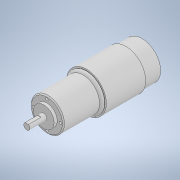
# Autodesk Inventor part: RS-555-71
Saved by Autodesk Inventor 2021 (Build 250183000, 183)
## iProperties
Created: 2022-02-01
Part Number: RS-555-71
Material: 一般
Document SubType Name: Modeling
Designer: hirohumi
Density: 1 g/cm^3
Appearance: 既定
Author: hirohumi
Autodesk Inventor part; units mm, degrees
ref_plane "YZ Plane" through (0, 0, 0) normal (1, 0, 0) x (0, 1, 0)
ref_plane "XZ Plane" through (0, 0, 0) normal (0, 1, 0) x (-1, 0, 0)
ref_plane "XY Plane" through (0, 0, 0) normal (0, 0, 1) x (1, 0, 0)
sketch "スケッチ1" plane through (0, 0, 0) normal (0, 0, 1) x (1, 0, 0)
  circle A0 centre (0, 0) radius 17.9
  dimension "d0" = 35.8
  constraints: 1 centre point, 1 coincident
  measures "d0" diameter of A0
extrude "押し出し1" add sketch "スケッチ1" against normal blind 3.3
fillet "フィレット1" radius 3 1 edges at (-17.9, 0, 0)
sketch "スケッチ2" plane through (0, 0, -3.3) normal (0, 0, -1) x (-1, 0, 0)
  circle A0 centre (0, 0) radius 19.25
  dimension "d4" = 38.5
  constraints: 1 centre point, 1 coincident
  measures "d4" diameter of A0
extrude "押し出し2" add sketch "スケッチ2" along normal blind 38
sketch "スケッチ3" plane through (0, 0, -41.3) normal (0, 0, -1) x (-1, 0, 0)
  circle A0 centre (0, 0) radius 17.9
  dimension "d7" = 35.8
  constraints: 1 centre point, 1 coincident
  measures "d7" diameter of A0
extrude "押し出し3" add sketch "スケッチ3" along normal blind 15.7
sketch "スケッチ4" plane through (0, 0, -57) normal (0, 0, -1) x (-1, 0, 0)
  circle A0 centre (0, 0) radius 1.585
  dimension "d10" = 3.17
  constraints: 1 centre point, 1 coincident
  measures "d10" diameter of A0
extrude "押し出し4" add sketch "スケッチ4" along normal blind 10.7
sketch "スケッチ5" plane through (0, 0, 0) normal (0, 0, 1) x (1, 0, 0)
  circle A0 centre (0, 0) radius 1.585 projected
  circle A1 centre (0, 0) radius 16
  dimension "d13" = 32
  constraints: 1 centre point, 1 coincident
  measures "d13" diameter of A1
extrude "押し出し5" add sketch "スケッチ5" along normal blind 34.9 contours A0 | A1
chamfer "面取り1" distance 1 angle 45 1 edges at (-16, 0, 34.9)
sketch "スケッチ6" plane through (0, 0, 34.9) normal (0, 0, 1) x (1, 0, 0)
  circle A0 centre (0, 0) radius 10
  dimension "d19" = 20
  constraints: 1 centre point, 1 coincident
  measures "d19" diameter of A0
extrude "押し出し6" add sketch "スケッチ6" along normal blind 3
sketch "スケッチ7" plane through (0, 0, 37.9) normal (0, 0, 1) x (1, 0, 0)
  circle A0 centre (0, 0) radius 1.585 projected
  circle A1 centre (0, 0) radius 3
  dimension "d22" = 6
  constraints: 1 centre point, 1 coincident
  measures "d22" diameter of A1
extrude "押し出し7" add sketch "スケッチ7" along normal blind 16.3 contours A0 | A1
sketch "スケッチ8" plane through (0, 0, 54.2) normal (0, 0, 1) x (1, 0, 0)
  circle A0 centre (0, 0) radius 3 projected
  line L0 (-1.6583, 2.5) -> (1.6583, 2.5)
  arc A1 (1.6583, 2.5) -> (-1.6583, 2.5) centre (0, 0) ccw
  dimension "d25" = 2.5
  constraints: 4 point on circle, 2 end point, 1 centre point, 1 coincident, 1 horizontal
  measures "d25" distance from line of point (0, 0) L0
extrude "押し出し8" cut sketch "スケッチ8" against normal blind 12 contours L0 A0 picked at (-0.1169, 2.6598)
sketch "スケッチ9" plane through (0, 0, 34.9) normal (0, 0, 1) x (1, 0, 0)
  circle A0 centre (0, 13) radius 1.25
  circle A1 centre (-13, 0) radius 1.25
  circle A2 centre (0, -13) radius 1.25
  circle A3 centre (13, 0) radius 1.25
  circle A4 centre (0, 0) radius 13 construction
  dimension "d28" = 2.5
  dimension "d29" = 2.5
  dimension "d30" = 2.5
  dimension "d31" = 2.5
  dimension "d32" = 26
  constraints: 5 centre point, 4 point on circle, 2 horizontal alignment, 2 vertical alignment, 1 coincident
  measures "d28" diameter of A0
  measures "d29" diameter of A1
  measures "d30" diameter of A2
  measures "d31" diameter of A3
  measures "d32" diameter of A4
extrude "押し出し9" cut sketch "スケッチ9" against normal blind 12
